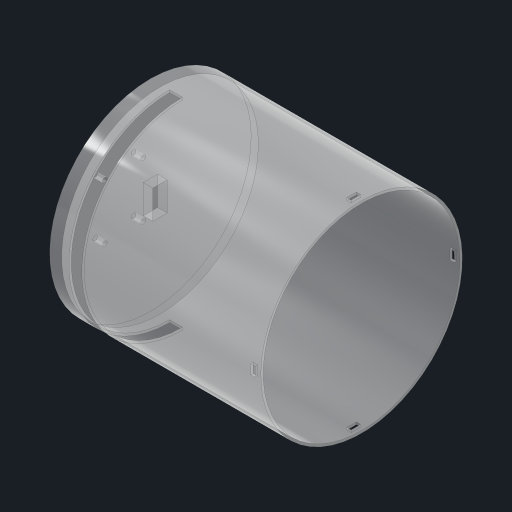
# Autodesk Inventor part: OUTK_001_ChipBucket
Saved by Autodesk Inventor 2024.2 (Build 282272000, 272)
## iProperties
Created: 2024-11-24
Part Number: OUTK_001_ChipBucket
Material: Polycarbonate, Clear
Document SubType Name: Modeling
Designer: Bryan
Density: 1.2 g/cm^3
Appearance: Polycarbonate - Clear
Author: Bryan
Autodesk Inventor part; units mm, degrees
ref_plane "YZ Plane" through (0, 0, 0) normal (1, 0, 0) x (0, 1, 0)
ref_plane "XZ Plane" through (0, 0, 0) normal (0, 1, 0) x (-1, 0, 0)
ref_plane "XY Plane" through (0, 0, 0) normal (0, 0, 1) x (1, 0, 0)
sketch "Sketch1" plane through (0, 0, 0) normal (1, 0, 0) x (0, 1, 0)
  circle A0 centre (0, 0) radius 133.35
  dimension "d0" = 266.7
  constraints: 1 centre point, 1 coincident
  measures "d0" diameter of A0
extrude "Extrusion1" add sketch "Sketch1" along normal mid plane 279.4
sketch "Sketch2" plane through (139.7, 0, 0) normal (1, 0, 0) x (0, 0, -1)
  circle A0 centre (0, 0) radius 130.175
  dimension "d3" = 260.35
  constraints: 1 centre point, 1 coincident
  measures "d3" diameter of A0
extrude "Extrusion2" cut sketch "Sketch2" against normal blind 266.7
sketch "Sketch3" plane through (0, 0, 0) normal (0, 0, 1) x (1, 0, 0)
  line L0 (-127, 130.175) -> (-127, -130.175) projected
  line L1 (139.7, 130.175) -> (139.7, -130.175) projected
  line L2 (139.7, 130.175) -> (-127, 130.175) projected
  line L3 (139.7, -130.175) -> (-127, -130.175) projected
  line L4 (-114.3, 130.175) -> (-114.3, -130.175)
  line L5 (-97.155, -130.175) -> (-97.155, 130.175)
  point P0 (0, 0)
  dimension "d6" = 12.7
  dimension "d7" = 17.145
  constraints: 4 end point, 4 point on line, 1 parallel, 1 vertical
  measures "d6" distance between parallel lines of L0 L4
  measures "d7" distance between parallel lines of L4 L5
extrude "Extrusion3" cut sketch "Sketch3" along normal blind 266.7 contours L2 L5 L3 L4
sketch "Sketch4" plane through (0, 0, 0) normal (0, 1, 0) x (-1, 0, 0)
  line L0 (114.3, 0) -> (97.155, 0) projected
  line L1 (114.3, 0) -> (114.3, 28.9256) projected
  line L2 (97.155, 0) -> (97.155, 28.9256) projected
  line L3 (97.155, 28.9256) -> (114.3, 28.9256) projected
  point P0 (0, 0)
extrude "Extrusion4" cut sketch "Sketch4" along normal through all both and the other way through all
sketch "Sketch5" plane through (0, 0, 0) normal (0, 1, 0) x (-1, 0, 0)
  line L0 (-126.365, 6.35) -> (-132.08, 6.35)
  line L1 (-132.08, 6.35) -> (-132.08, -6.35)
  line L2 (-132.08, -6.35) -> (-126.365, -6.35)
  line L3 (-126.365, -6.35) -> (-126.365, 6.35)
  line L4 (-139.7, 133.35) -> (-139.7, -133.35) projected
  point P0 (0, 0)
  point P1 (-126.365, 0)
  dimension "d12" = 5.715
  dimension "d13" = 12.7
  dimension "d14" = 7.62
  constraints: 8 end point, 2 parallel, 1 horizontal, 1 horizontal alignment, 1 midpoint, 1 perpendicular
  measures "d12" distance of L2.end L1.end
  measures "d13" distance of L1.end L0.end
  measures "d14" distance between parallel lines of L4 L1
extrude "Extrusion5" cut sketch "Sketch5" along normal through all both and the other way through all
sketch "Sketch6" plane through (0, 0, 0) normal (0, 0, 1) x (1, 0, 0)
  line L0 (126.365, 6.35) -> (132.08, 6.35)
  line L1 (132.08, 6.35) -> (132.08, -6.35)
  line L2 (132.08, -6.35) -> (126.365, -6.35)
  line L3 (126.365, -6.35) -> (126.365, 6.35)
  line L4 (139.7, -133.35) -> (139.7, 133.35) projected
  point P0 (0, 0)
  point P1 (126.365, 0)
  dimension "d17" = 5.715
  dimension "d18" = 12.7
  dimension "d19" = 7.62
  constraints: 8 end point, 2 parallel, 1 horizontal, 1 horizontal alignment, 1 midpoint, 1 perpendicular
  measures "d17" distance of L1.end L2.end
  measures "d18" distance of L0.end L1.end
  measures "d19" distance between parallel lines of L4 L1
extrude "Extrusion6" cut sketch "Sketch6" along normal through all both and the other way through all
sketch "Sketch8" plane through (-139.7, 0, 0) normal (-1, 0, 0) x (0, 0, 1)
  line L0 (-9.525, -19.05) -> (9.525, -19.05)
  line L1 (9.525, -19.05) -> (9.525, 19.05)
  line L2 (9.525, 19.05) -> (-9.525, 19.05)
  line L3 (-9.525, 19.05) -> (-9.525, -19.05)
  line L4 (-9.525, -19.05) -> (9.525, 19.05) construction
  line L5 (9.525, -19.05) -> (-9.525, 19.05) construction
  circle A0 centre (22.225, 60) radius 3.2512
  circle A1 centre (22.225, -12.7) radius 3.2512
  circle A2 centre (73.025, 60) radius 3.2512
  circle A3 centre (73.025, -12.7) radius 3.2512
  point P0 (0, 0)
  dimension "d22" = 19.05
  dimension "d23" = 38.1
  dimension "d24" = 6.5024
  dimension "d25" = 72.7
  dimension "d26" = 50.8
  dimension "d27" = 12.7
  dimension "d28" = 12.7
  constraints: 12 end point, 4 centre point, 3 equal radius, 2 horizontal alignment, 2 midpoint, 2 parallel, 2 vertical alignment, 1 horizontal, 1 perpendicular
  measures "d22" distance of L2.end L1.end
  measures "d23" distance of L1.end L0.end
  measures "d24" diameter of A0
  measures "d25" distance of A3.centre A2.centre
  measures "d26" distance of A3.centre A1.centre
  measures "d27" vertical distance of point (0, 0) A1.centre
  measures "d28" distance from line of A1.centre L1
extrude "Extrusion7" cut sketch "Sketch8" against normal blind 25.4
body "Solid1"
